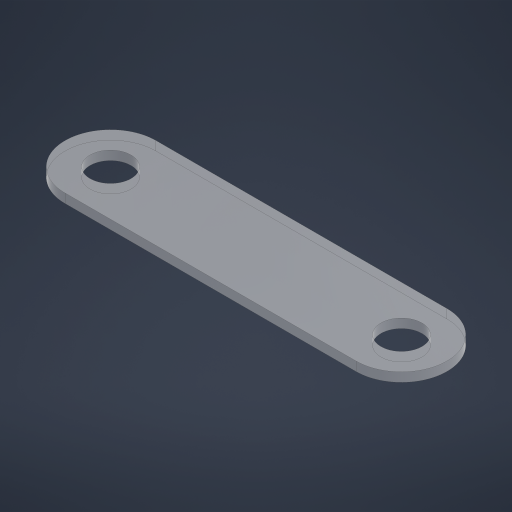
# Autodesk Inventor part: CORL_006_SmallPlate
Saved by Autodesk Inventor 2024.2 (Build 282272000, 272)
## iProperties
Created: 2024-08-02
Part Number: CORL_006_SmallPlate
Material: Polycarbonate, Clear
Document SubType Name: Modeling
Designer: Bryan
Density: 1.2 g/cm^3
Appearance: Polycarbonate - Clear
Author: Bryan
Autodesk Inventor part; units mm, degrees
ref_plane "YZ Plane" through (0, 0, 0) normal (1, 0, 0) x (0, 1, 0)
ref_plane "XZ Plane" through (0, 0, 0) normal (0, 1, 0) x (-1, 0, 0)
ref_plane "XY Plane" through (0, 0, 0) normal (0, 0, 1) x (1, 0, 0)
sketch "Sketch1" plane through (0, 0, 0) normal (0, 1, 0) x (-1, 0, 0)
  circle A0 centre (0, 0) radius 14.2875
  line L0 (0, 0) -> (203.2, 0) construction
  circle A1 centre (203.2, 0) radius 14.2875
  circle A2 centre (0, 0) radius 31.75 construction
  circle A3 centre (203.2, 0) radius 31.75 construction
  line L1 (203.2, -31.75) -> (0, -31.75)
  line L2 (0, 31.75) -> (203.2, 31.75)
  arc A4 (203.2, -31.75) -> (203.2, 31.75) centre (203.2, 0) ccw
  arc A5 (0, 31.75) -> (0, -31.75) centre (0, 0) ccw
  dimension "d0" = 28.575
  dimension "d1" = 203.2
  dimension "d2" = 63.5
  constraints: 8 point on circle, 7 tangent, 6 centre point, 6 end point, 4 coincident, 2 equal radius, 1 horizontal
  measures "d0" diameter of A0
  measures "d1" distance of L0.start L0.end
  measures "d2" diameter of A2
extrude "Extrusion1" add sketch "Sketch1" along normal blind 6.35
body "Solid1"
